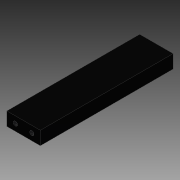
# Autodesk Inventor part: Fixture_Base_Support-02
Saved by Autodesk Inventor 2015 (Build 190159000, 159)
## iProperties
Created: 2014-12-16
Part Number: Fixture_Base_Support-02
Material: Generic
Document SubType Name: Modeling
Designer: amarschn
Density: 1 g/cm^3
Appearance: Anodized - Black
Author: amarschn
Autodesk Inventor part; units mm, degrees
ref_plane "YZ Plane" through (0, 0, 0) normal (1, 0, 0) x (0, 1, 0)
ref_plane "XZ Plane" through (0, 0, 0) normal (0, 1, 0) x (-1, 0, 0)
ref_plane "XY Plane" through (0, 0, 0) normal (0, 0, 1) x (1, 0, 0)
sketch "Sketch1" plane through (0, 0, 0) normal (0, 1, 0) x (-1, 0, 0)
  line L0 (-15.5575, -61.7537) -> (15.5575, -61.7537)
  line L1 (15.5575, -61.7537) -> (15.5575, 61.7538)
  line L2 (15.5575, 61.7538) -> (-15.5575, 61.7538)
  line L3 (-15.5575, 61.7538) -> (-15.5575, -61.7537)
  line L4 (-15.5575, -61.7537) -> (15.5575, 61.7538) construction
  line L5 (15.5575, -61.7537) -> (-15.5575, 61.7538) construction
  point P0 (0, 0)
  dimension "d0" = 123.5075
  dimension "d1" = 31.115
  constraints: 12 end point, 2 midpoint, 2 parallel, 1 horizontal, 1 perpendicular
  measures "d0" distance of L0.end L1.end
  measures "d1" distance of L0.start L0.end
extrude "Extrusion1" add sketch "Sketch1" along normal blind 12.446
sketch "Sketch2" plane through (-15.5575, 0, 61.7538) normal (0, 0, 1) x (1, 0, 0)
  line L0 (15.5575, 17.8749) -> (15.5575, -12.6883)
  line L1 (35.533, 6.223) -> (0.122, 6.223)
  line L2 (0, 0) -> (31.115, 0) projected
  line L3 (31.115, 0) -> (31.115, 12.446) projected
  point P0 (15.5575, 0)
  point P1 (15.5575, 0)
  point P2 (15.5575, 0)
  point P3 (31.115, 6.223)
  point P4 (7.9375, 6.223)
  point P5 (23.1775, 6.223)
  dimension "d4" = 15.24
  constraints: 4 end point, 4 midpoint, 3 point on line, 1 horizontal, 1 symmetric about line, 1 vertical
  measures "d4" distance of point (23.178, 6.223) point (7.938, 6.223)
hole "Hole1" at (-7.62, 6.223, 61.7538) at (7.62, 6.223, 61.7538) direction (0, 0, -1) diameter 3.9624 depth 17.78 tip angle 118 thread size "10-32 UNF" class "2B" standard "ANSI Unified Screw Threads"
ref_plane "Work Plane2" through (15.5575, 0, 0) normal (0, 0, -1) x (-1, 0, 0)
mirror "Mirror1" about plane through (15.5575, 0, 0) normal (0, 0, -1) of "Hole1"
body "Solid1"
